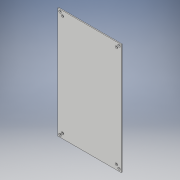
# Autodesk Inventor part: Grundplatte
Saved by Autodesk Inventor 2017 (Build 210142000, 142)
## iProperties
Part Number: Grundplatte
Material: Generisch
Document SubType Name: Modeling
Designer: Dima
Density: 1 g/cm^3
Appearance: Vorgabe
Author: Dima
Autodesk Inventor part; units mm, degrees
ref_plane "YZ Plane" through (0, 0, 0) normal (1, 0, 0) x (0, 1, 0)
ref_plane "XZ Plane" through (0, 0, 0) normal (0, 1, 0) x (-1, 0, 0)
ref_plane "XY Plane" through (0, 0, 0) normal (0, 0, 1) x (1, 0, 0)
sketch "Skizze1" plane through (0, 0, 0) normal (0, 1, 0) x (-1, 0, 0)
  line L0 (132.5635, 175.274) -> (-67.4365, 175.274)
  line L1 (-67.4365, 175.274) -> (-67.4365, -174.726)
  line L2 (-67.4365, -174.726) -> (132.5635, -174.726)
  line L3 (132.5635, -174.726) -> (132.5635, 175.274)
  line L4 (354.7243, 0.274) -> (-224.9528, 0.274)
  point P0 (0, 0)
  dimension "d0" = 350
  dimension "d1" = 200
  dimension "d2" = 175
  dimension "d3" = 175
  constraints: 10 end point, 2 horizontal, 2 parallel, 1 perpendicular
  measures "d0" distance of L2.end L0.start
  measures "d1" distance of L0.start L0.end
  measures "d2" distance between parallel lines of L0 L4
  measures "d3" distance between parallel lines of L2 L4
extrude "Extrusion1" add sketch "Skizze1" along normal blind 3
sketch "Skizze13" plane through (0, 0, 0) normal (0, -1, 0) x (1, 0, 0)
  line L0 (67.4365, 175.274) -> (67.4365, -174.726) construction
  line L1 (-132.5635, 175.274) -> (67.4365, 175.274) construction
  line L2 (-132.5635, -174.726) -> (-132.5635, 175.274) construction
  line L3 (67.4365, -174.726) -> (-132.5635, -174.726) construction
  point P0 (0, 0)
  point P1 (-125.5635, -167.726)
  point P2 (-117.5635, -159.726)
  point P3 (-125.5635, 168.274)
  point P4 (-117.5635, 160.274)
  point P5 (52.4365, 160.274)
  point P6 (60.4365, 168.274)
  point P7 (60.4365, -167.726)
  point P8 (52.4365, -159.726)
  dimension "d131" = 7
  dimension "d132" = 7
  dimension "d133" = 15
  dimension "d134" = 15
  dimension "d135" = 7
  dimension "d136" = 7
  dimension "d137" = 7
  dimension "d138" = 7
  dimension "d140" = 7
  dimension "d141" = 15
  dimension "d142" = 15
  dimension "d143" = 15
  dimension "d144" = 15
  dimension "d146" = 15
  measures "d131" distance from line of point (-125.564, -167.726) L3
  measures "d132" distance from line of L2 point (-125.564, -167.726)
  measures "d133" distance from line of L3 point (-117.564, -159.726)
  measures "d134" distance from line of L2 point (-117.564, -159.726)
  measures "d135" distance from line of L1 point (-125.564, 168.274)
  measures "d136" distance from line of L2 point (-125.564, 168.274)
  measures "d137" distance from line of L1 point (60.436, 168.274)
  measures "d138" distance from line of L0 point (60.436, 168.274)
  measures "d140" distance from line of L3 point (60.436, -167.726)
  measures "d141" distance from line of L1 point (-117.564, 160.274)
  measures "d142" distance from line of L2 point (-117.564, 160.274)
  measures "d143" distance from line of L0 point (52.436, 160.274)
  measures "d144" distance from line of L1 point (52.436, 160.274)
  measures "d146" distance from line of L3 point (52.436, -159.726)
hole "Bohrung2" at (60.4365, 0, -167.726) at (52.4365, 0, -159.726) at (-117.5635, 0, -159.726) at (-125.5635, 0, -167.726) at (-117.5635, 0, 160.274) at (-125.5635, 0, 168.274) at (52.4365, 0, 160.274) at (60.4365, 0, 168.274) direction (0, 1, 0) diameter 4.5 end through all countersink diameter 8 countersink angle 90
equation "\"d132\" = d131"
equation "\"d134\" = d133"
equation "\"d135\" = d131"
equation "\"d136\" = d131"
equation "\"d137\" = d131"
equation "\"d138\" = d131"
equation "\"d140\" = d131"
equation "\"d141\" = d133"
equation "\"d142\" = d133"
equation "\"d143\" = d133"
equation "\"d144\" = d133"
